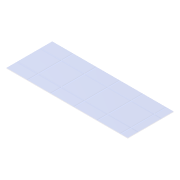
# Autodesk Inventor part: HousingCage_Sidepanel_short
Saved by Autodesk Inventor 2016 (Build 200138000, 138)
## iProperties
Created: 2012-11-26
Part Number: HousingCage_Sidepanel_short
Material: PMMA Plastic
Document SubType Name: Modeling
Designer: Neef
Mass: 280.023 g
Surface Area: 1611.83 cm^2
Volume: 235.71 cm^3
Density: 1.188 g/cm^3
Appearance: Polycarbonate - Clear
Author: Neef
Autodesk Inventor part; units mm, degrees
ref_plane "YZ Plane" through (0, 0, 0) normal (1, 0, 0) x (0, 1, 0)
ref_plane "XZ Plane" through (0, 0, 0) normal (0, 1, 0) x (-1, 0, 0)
ref_plane "XY Plane" through (0, 0, 0) normal (0, 0, 1) x (1, 0, 0)
sketch "Skizze1" plane through (0, 0, 0) normal (0, 0, 1) x (1, 0, 0)
  line L0 (0, 140) -> (0, -140) projected
  line L1 (-370.86, 0) -> (370.86, 0) projected
  line L2 (264.9, 100) -> (-264.9, 100)
  line L3 (-264.9, 100) -> (-264.9, -100)
  line L4 (-264.9, -100) -> (264.9, -100)
  line L5 (264.9, -100) -> (264.9, 100)
  point P0 (0, 0)
  point P1 (264.9, 0)
  point P2 (0, 100)
  dimension "d0" = 200
  dimension "d1" = 529.8
  constraints: 8 end point, 2 midpoint, 2 parallel, 2 point on line, 1 horizontal, 1 perpendicular
  measures "d0" distance of L4.end L2.start
  measures "d1" distance of L2.start L2.end
extrude "Extrusion1" add sketch "Skizze1" along normal blind 3
